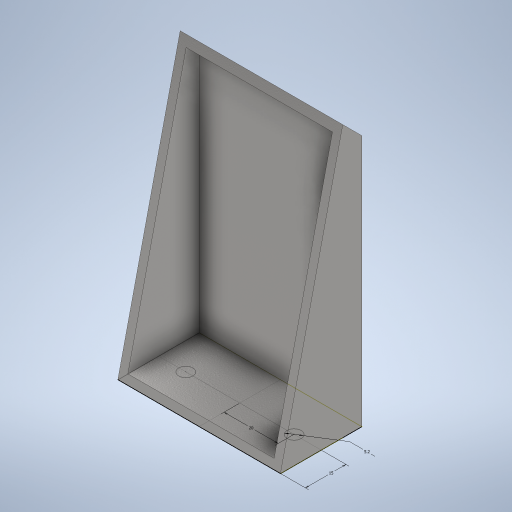
# Autodesk Inventor part: Claw
Saved by Autodesk Inventor 2024.2 (Build 282272000, 272)
## iProperties
Created: 2025-04-11
Part Number: Claw
Material: Generic
Document SubType Name: Modeling
Designer: Admin
Density: 1 g/cm^3
Appearance: Galvanized
Author: Admin
Autodesk Inventor part; units mm, degrees
ref_plane "YZ Plane" through (0, 0, 0) normal (1, 0, 0) x (0, 1, 0)
ref_plane "XZ Plane" through (0, 0, 0) normal (0, 1, 0) x (-1, 0, 0)
ref_plane "XY Plane" through (0, 0, 0) normal (0, 0, 1) x (1, 0, 0)
sketch "Sketch4" plane through (0, 0, 0) normal (0, 1, 0) x (-1, 0, 0)
  line L0 (0, 0) -> (60, 0)
  line L1 (60, 0) -> (60, -30)
  line L2 (60, -30) -> (0, -30)
  line L3 (0, -30) -> (0, 0)
  dimension "d15" = 60
  dimension "d16" = 30
  constraints: 8 end point, 2 parallel, 1 horizontal, 1 perpendicular
  measures "d15" distance of L1.end L2.end
  measures "d16" distance of L0.end L1.end
extrude "Extrusion4" add sketch "Sketch4" along normal blind 100
chamfer "Chamfer1" distance 7 angle 45 1 edges at (-30, 100, -30)
sketch "Sketch6" plane through (0, 0, 0) normal (1, 0, 0) x (0, 0, -1)
  line L0 (30, 0) -> (30, 93) projected
  line L1 (0, 0) -> (0, 100) projected
  line L2 (30, 0) -> (0, 0)
  line L3 (0, 0) -> (0, 100)
  line L4 (0, 100) -> (30, 100)
  line L5 (30, 100) -> (30, 0)
  line L6 (0, 0) -> (23.0011, 100)
  constraints: 10 end point, 2 parallel, 1 horizontal, 1 perpendicular, 1 point on line
extrude "Extrusion5" cut sketch "Sketch6" against normal blind 100 contours L1 L4 L6
shell "Shell2" thickness 3 removed faces 1 at (-40, 66.6661, -15.3339)
sketch "Sketch8" plane through (0, 0, 0) normal (0, -1, 0) x (1, 0, 0)
  line L0 (0, -30) -> (-60, -30) projected
  line L1 (0, 0) -> (-60, 0)
  line L2 (-60, 0) -> (-60, -30)
  line L3 (-60, -30) -> (0, -30)
  line L4 (0, -30) -> (0, 0)
  line L5 (0, -23.0009) -> (0, 0) projected
  line L6 (0, 0) -> (0, -15)
  line L7 (0, -15) -> (-60, -15) construction
  line L8 (-30, 0) -> (-30, -30) construction
  line L9 (-30, -15) -> (-10, -15) construction
  circle A0 centre (-10, -15) radius 2.6
  line L10 (-30, -15) -> (-50, -15) construction
  circle A1 centre (-50, -15) radius 2.6
  dimension "d26" = 15
  dimension "d27" = 20
  dimension "d28" = 5.2
  constraints: 18 end point, 4 midpoint, 2 centre point, 2 coincident, 2 parallel, 2 point on line, 2 symmetric about line, 1 horizontal, 1 perpendicular, 1 other
  measures "d26" distance of L1.start L6.end
  measures "d27" distance of L9.start L9.end
  measures "d28" diameter of A0
body "Solid2"
